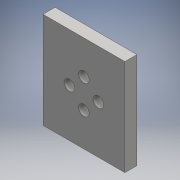
# Autodesk Inventor part: cameraMount
Saved by Autodesk Inventor 2016 (Build 200138000, 138)
## iProperties
Created: 2016-05-02
Part Number: cameraMount
Material: Generic
Document SubType Name: Modeling
Designer: mkepler
Density: 1 g/cm^3
Appearance: Default
Author: mkepler
Autodesk Inventor part; units mm, degrees
ref_plane "YZ Plane" through (0, 0, 0) normal (1, 0, 0) x (0, 1, 0)
ref_plane "XZ Plane" through (0, 0, 0) normal (0, 1, 0) x (-1, 0, 0)
ref_plane "XY Plane" through (0, 0, 0) normal (0, 0, 1) x (1, 0, 0)
sketch "Sketch1" plane through (0, 0, 0) normal (0, 1, 0) x (-1, 0, 0)
  line L0 (0, 0) -> (34, 0)
  line L1 (34, 0) -> (34, -40)
  line L2 (34, -40) -> (0, -40)
  line L3 (0, -40) -> (0, 0)
  line L4 (17, -40) -> (17, 0)
  line L5 (34, -20) -> (0, -20)
  dimension "d0" = 34
  dimension "d1" = 40
  constraints: 12 end point, 4 midpoint, 2 parallel, 1 horizontal, 1 perpendicular
  measures "d0" distance of L1.end L2.end
  measures "d1" distance of L0.end L1.end
extrude "Extrusion1" add sketch "Sketch1" along normal blind 3
sketch "Sketch2" plane through (0, 3, 0) normal (0, 1, 0) x (1, 0, 0)
  line L0 (-34, 40) -> (-34, 0) projected
  line L1 (0, 0) -> (0, 40) projected
  line L2 (0, 40) -> (-34, 40) projected
  line L3 (-34, 0) -> (0, 0) projected
  circle A0 centre (-17, 20) radius 9
  line L4 (-34, 0) -> (0, 0)
  line L5 (0, 0) -> (0, 40)
  line L6 (0, 40) -> (-34, 40)
  line L7 (-34, 40) -> (-34, 0)
  dimension "d4" = 18
  constraints: 8 end point, 2 parallel, 1 centre point, 1 horizontal, 1 perpendicular
  measures "d4" diameter of A0
extrude "Extrusion2" add sketch "Sketch2" along normal blind 2
sketch "Sketch4" plane through (-17, 3, -20) normal (0, 1, 0) x (1, 0, 0)
  line L0 (0, 0) -> (0, 6)
  circle A0 centre (0, 6) radius 2.175
  circle A1 centre (0, -6) radius 2.175
  circle A2 centre (6, 0) radius 2.175
  circle A3 centre (-6, 0) radius 2.175
  point P0 (17, -20)
  dimension "d7" = 6
  dimension "d8" = 4.35
  dimension "d9" = 4.35
  dimension "d10" = 12
  dimension "d11" = 4.35
  dimension "d12" = 6
  dimension "d13" = 4.35
  dimension "d14" = 12
  constraints: 4 centre point, 2 end point, 1 coincident, 1 vertical
  measures "d7" distance of L0.start L0.end
  measures "d8" diameter of A0
  measures "d9" diameter of A1
  measures "d10" distance of L0.end A1.centre
  measures "d11" diameter of A2
  measures "d12" distance of L0.start A2.centre
  measures "d13" diameter of A3
  measures "d14" distance of A2.centre A3.centre
hole "Hole1" at (-23, 3, -20) at (-17, 3, -26) at (-11, 3, -20) at (-17, 3, -14) direction (0, -1, 0) diameter 4.35 end through all
body "Solid1"
